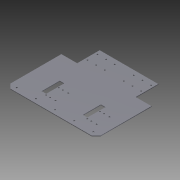
# Autodesk Inventor part: Chasis
Saved by Autodesk Inventor 2014 (Build 180170000, 170)
## iProperties
Created: 2014-01-26
Part Number: Chasis
Material: Acero dulce
Document SubType Name: Chapa
Designer: VICTOR
Density: 7.86 g/cm^3
Sheet Metal Rule: Por defecto_mm
Mass: 380.435 g
Surface Area: 660.124 cm^2
Volume: 48.4014 cm^3
Sheet Metal Width: 0,000 mm
Sheet Metal Length: 0,000 mm
Sheet Metal Area: 0,000 mm^2
Project: ROBOT SUMO
Description: CHASIS
Appearance: Acero
Author: Sanjo
Revision Number: 1
Autodesk Inventor part; units mm, degrees
ref_plane "YZ Plane" through (0, 0, 0) normal (1, 0, 0) x (0, 1, 0)
ref_plane "XZ Plane" through (0, 0, 0) normal (0, 1, 0) x (-1, 0, 0)
ref_plane "XY Plane" through (0, 0, 0) normal (0, 0, 1) x (1, 0, 0)
sketch "Boceto1" plane through (0, 0, 0) normal (0, 0, 1) x (1, 0, 0)
  line L0 (-100, 105) -> (100, 105)
  line L1 (100, 105) -> (100, -68)
  line L2 (100, -68) -> (-100, -68)
  line L3 (-100, -68) -> (-100, 105)
  point P0 (0, 0)
  dimension "d0" = 200
  dimension "d1" = 173
  dimension "d2" = 100
  dimension "d127" = 105
  measures "d0" distance of L1.end L2.end
  measures "d1" distance of L0.end L1.end
  measures "d2" distance from line of point (0, 0) L1
  measures "d127" distance from line of L0 point (0, 0)
extrude "Placa1" add sketch "Boceto1" along normal blind 1.5
sketch "Boceto2" plane through (0, 0, 1.5) normal (0, 0, 1) x (1, 0, 0)
  line L0 (100, 105) -> (100, -68)
  line L1 (-100, 105) -> (100, 105)
  line L2 (-100, -68) -> (-100, 105)
  line L3 (100, -68) -> (-100, -68)
  line L4 (-100, 55) -> (-65, 55)
  line L5 (-65, 55) -> (-65, 105)
  line L6 (100, 55) -> (65, 55)
  line L7 (65, 55) -> (65, 105)
  line L8 (-100, 105) -> (-100, 55)
  line L9 (100, 55) -> (100, 105)
  point P0 (0, 0)
  point P1 (-100, 65)
  point P2 (100, 65)
  dimension "d6" = 50
  dimension "d9" = 50
  dimension "d52" = 35
  dimension "d58" = 35
  constraints: 20 end point, 6 point on line, 2 parallel, 2 perpendicular
  measures "d6" distance between parallel lines of L1 L4
  measures "d9" distance between parallel lines of L1 L6
  measures "d52" distance between parallel lines of L0 L7
  measures "d58" distance between parallel lines of L2 L5
extrude "Cortar3" cut sketch "Boceto2" against normal blind 1.5 contours L0 L6 L7 L1 | L5 L4 L2 L1
chamfer "Chaflán de esquina1" distance 10 angle 45 2 edges at (100, -68, 0.75) (-100, -68, 0.75)
sketch "Boceto9" plane through (0, 0, 0) normal (0, 0, -1) x (-1, 0, 0)
  point P0 (43.7, 83.5)
sketch "Boceto10" plane through (0, 0, 0) normal (0, 0, -1) x (-1, 0, 0)
  point P0 (5.3, 83.5)
sketch "Boceto11" plane through (0, 0, 0) normal (0, 0, -1) x (-1, 0, 0)
  point P0 (-43.7, 83.5)
sketch "Boceto12" plane through (0, 0, 0) normal (0, 0, -1) x (-1, 0, 0)
  point P0 (-5.3, 83.5)
sketch "Boceto18" plane through (0, 0, 0) normal (0, 0, -1) x (-1, 0, 0)
  point P0 (-42.5, -59)
  point P1 (42.5, -59)
  point P2 (85, -59)
  point P3 (0, -59)
  point P4 (-85, -59)
hole "Hole16" at (42.5, -59, 0) at (-42.5, -59, 0) at (-85, -59, 0) at (0, -59, 0) at (85, -59, 0) direction (0, 0, 1) diameter 3.2 depth 1.5
sketch "Boceto21" plane through (0, 0, 1.5) normal (0, 0, 1) x (1, 0, 0)
  circle A0 centre (59.5, 72.5) radius 1.5
  circle A1 centre (59.5, 94.5) radius 1.5
  circle A2 centre (40.3, 72.5) radius 1.5
  circle A3 centre (40.3, 94.5) radius 1.5
  circle A4 centre (21.1, 72.5) radius 1.5
  circle A5 centre (21.1, 94.5) radius 1.5
  circle A6 centre (-59.5, 72.5) radius 1.5
  circle A7 centre (-59.5, 94.5) radius 1.5
  circle A8 centre (-40.3, 72.5) radius 1.5
  circle A9 centre (-40.3, 94.5) radius 1.5
  circle A10 centre (-21.1, 72.5) radius 1.5
  circle A11 centre (-21.1, 94.5) radius 1.5
  point P0 (0, 0)
  dimension "d151" = 3
  dimension "d152" = 3
  dimension "d153" = 3
  dimension "d154" = 3
  dimension "d155" = 3
  dimension "d156" = 3
  constraints: 12 centre point
  measures "d151" diameter of A0
  measures "d152" diameter of A1
  measures "d153" diameter of A2
  measures "d154" diameter of A3
  measures "d155" diameter of A4
  measures "d156" diameter of A5
hole "Hole17" at (-59.5, 94.5, 1.5) at (-59.5, 72.5, 1.5) at (-40.3, 94.5, 1.5) at (-40.3, 72.5, 1.5) at (-21.1, 94.5, 1.5) at (-21.1, 72.5, 1.5) at (21.1, 94.5, 1.5) at (21.1, 72.5, 1.5) at (59.5, 94.5, 1.5) at (59.5, 72.5, 1.5) at (40.3, 72.5, 1.5) at (40.3, 94.5, 1.5) direction (0, 0, -1) diameter 3 end through all
sketch "Boceto20" plane through (0, 0, 1.5) normal (0, 0, 1) x (1, 0, 0)
  line L0 (-50.6711, 2.0067) -> (-40.6711, 2.0067)
  line L1 (-40.6711, 2.0067) -> (-40.6711, -37.9933)
  line L2 (-40.6711, -37.9933) -> (-50.6711, -37.9933)
  line L3 (-50.6711, -37.9933) -> (-50.6711, 2.0067)
  line L4 (50.6711, 2.0067) -> (40.6711, 2.0067)
  line L5 (40.6711, 2.0067) -> (40.6711, -37.9933)
  line L6 (40.6711, -37.9933) -> (50.6711, -37.9933)
  line L7 (50.6711, -37.9933) -> (50.6711, 2.0067)
  point P0 (0, 0)
  dimension "d171" = 10
  dimension "d172" = 40
  dimension "d190" = 40.6711
  dimension "d191" = 40.6711
  dimension "d192" = 40
  dimension "d193" = 10
  constraints: 16 end point, 2 parallel, 1 horizontal, 1 perpendicular
  measures "d171" distance of L1.end L2.end
  measures "d172" distance of L2.end L0.start
  measures "d190" horizontal distance of point (0, 0) L0.end
  measures "d191" distance from line of L5 point (0, 0)
  measures "d192" distance of L5.start L5.end
  measures "d193" distance of L5.end L6.end
extrude "Cortar6" cut sketch "Boceto20" against normal blind 1.5
sketch "Boceto22" plane through (0, 0, 1.5) normal (0, 0, 1) x (1, 0, 0)
  circle A0 centre (-29.2523, -12.388) radius 1.5
  circle A1 centre (-29.2523, -40.7295) radius 1.5
  circle A2 centre (-17.3656, -12.388) radius 1.5
  circle A3 centre (-17.3656, -40.7295) radius 1.5
  circle A4 centre (-38.1789, -12.388) radius 1.5
  circle A5 centre (-38.1789, -40.7295) radius 1.5
  circle A6 centre (62.09, -12.388) radius 1.5
  circle A7 centre (62.09, -40.7295) radius 1.5
  circle A8 centre (73.9767, -12.388) radius 1.5
  circle A9 centre (73.9767, -40.7295) radius 1.5
  circle A10 centre (53.1633, -12.388) radius 1.5
  circle A11 centre (53.1633, -40.7295) radius 1.5
  line L0 (50.6711, 2.0067) -> (50.6711, -37.9933) projected
  line L1 (-40.6711, 2.0067) -> (-40.6711, -37.9933) projected
  point P0 (0, 0)
  dimension "d175" = 3
  dimension "d176" = 3
  dimension "d177" = 3
  dimension "d178" = 3
  dimension "d186" = 3
  dimension "d187" = 3
  dimension "d188" = 3
  dimension "d189" = 3
  dimension "d194" = 11.8867
  dimension "d195" = 8.9267
  dimension "d196" = 2.4922
  dimension "d197" = 8.9267
  dimension "d198" = 11.8867
  dimension "d200" = 28.3415
  dimension "d201" = 8.9267
  dimension "d202" = 11.8867
  dimension "d203" = 8.9267
  dimension "d204" = 11.8867
  dimension "d205" = 28.3415
  dimension "d207" = 2.4922
  constraints: 12 centre point
  measures "d175" diameter of A0
  measures "d176" diameter of A1
  measures "d177" diameter of A2
  measures "d178" diameter of A3
  measures "d186" diameter of A6
  measures "d187" diameter of A7
  measures "d188" diameter of A8
  measures "d189" diameter of A9
  measures "d194" distance of A2.centre A0.centre
  measures "d195" distance of A0.centre A4.centre
  measures "d196" distance from line of L1 A4.centre
  measures "d197" distance of A1.centre A5.centre
  measures "d198" distance of A3.centre A1.centre
  measures "d200" distance of A3.centre A2.centre
  measures "d201" distance of A6.centre A10.centre
  measures "d202" distance of A8.centre A6.centre
  measures "d203" distance of A7.centre A11.centre
  measures "d204" distance of A9.centre A7.centre
  measures "d205" distance of A9.centre A8.centre
  measures "d207" distance from line of L0 A10.centre
hole "Hole18" at (-29.2523, -12.388, 1.5) at (-17.3656, -12.388, 1.5) at (-29.2523, -40.7295, 1.5) at (-17.3656, -40.7295, 1.5) at (-38.1789, -12.388, 1.5) at (-38.1789, -40.7295, 1.5) at (53.1633, -12.388, 1.5) at (62.09, -12.388, 1.5) at (53.1633, -40.7295, 1.5) at (62.09, -40.7295, 1.5) at (73.9767, -12.388, 1.5) at (73.9767, -40.7295, 1.5) direction (0, 0, -1) diameter 3 end through all
equation "\"d59\" = Grosor"
equation "\"d169\" = Grosor"
equation "\"d149\" = Grosor"
equation "\"d184\" = Grosor"
equation "\"Radio_pliegue\" = Grosor"
equation "\"Anchura_desahogo_plegado\" = Grosor"
equation "\"Profundidad_desahogo_plegado\" = 0.5 * Grosor"
equation "\"Tamaño_destalonado\" = 4 * Grosor"
equation "\"Remanente_mínimo\" = 2 * Grosor"
equation "\"Radiodetransición\" = Radio_pliegue"
equation "\"Tamaño_de_radio_de_Jacobi\" = Radio_pliegue"
equation "\"TamañoSeparación\" = Grosor"
equation "\"d4\" = Radio_pliegue"
equation "\"Grosor\" = 1.5"
